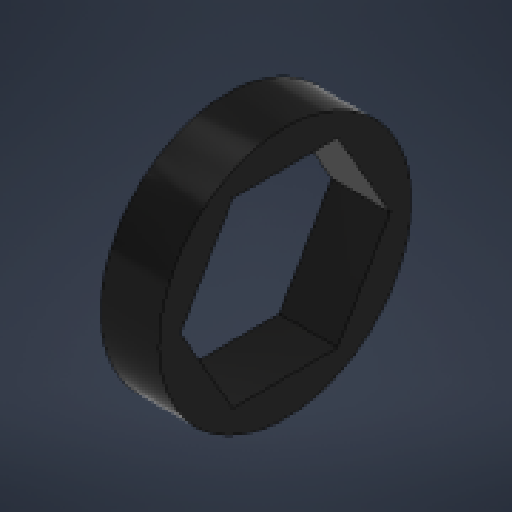
# Autodesk Inventor part: 3DPRINT,BACKROLLERS,INTERROLLER,SPACER
Saved by Autodesk Inventor 2026.1 (Build 301233020, 233B)
## iProperties
Created: 2026-01-27
Part Number: 3DPRINT,BACKROLLERS,INTERROLLER,SPACER
Material: ABS Plastic
Document SubType Name: Modeling
Designer: Owen L
Mass: 1.54469 g
Surface Area: 15.1586 cm^2
Volume: 1.45725 cm^3
Density: 1.06 g/cm^3
Appearance: Smooth - Black
Author: Owen L
Autodesk Inventor part; units mm, degrees
ref_plane "YZ Plane" through (0, 0, 0) normal (1, 0, 0) x (0, 1, 0)
ref_plane "XZ Plane" through (0, 0, 0) normal (0, 1, 0) x (-1, 0, 0)
ref_plane "XY Plane" through (0, 0, 0) normal (0, 0, 1) x (1, 0, 0)
sketch "Sketch1" plane through (0, 0, 0) normal (1, 0, 0) x (0, 1, 0)
  line L0 (-6.4135, -3.7028) -> (-6.4135, 3.7028)
  line L1 (-6.4135, 3.7028) -> (0, 7.4057)
  line L2 (0, 7.4057) -> (6.4135, 3.7028)
  line L3 (6.4135, 3.7028) -> (6.4135, -3.7028)
  line L4 (6.4135, -3.7028) -> (0, -7.4057)
  line L5 (0, -7.4057) -> (-6.4135, -3.7028)
  circle A0 centre (0, 0) radius 8.89
  dimension "d0" = 12.827
  dimension "d1" = 17.78
  constraints: 12 end point, 2 coincident, 1 centre point, 1 vertical, 13 other
  measures "d0" distance between parallel lines of L3 L0
  measures "d1" diameter of A0
extrude "Extrusion1" add sketch "Sketch1" along normal blind 4.1173
body "Solid1"
